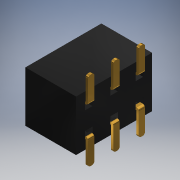
# Autodesk Inventor part: CON-IDC-HE-SMD-2X3-P2MM
Saved by Autodesk Inventor 2018.3 (Build 223284000, 284)
## iProperties
Created: 2020-10-20
Part Number: CON-IDC-HE-SMD-2X3-P2MM
Material: Genérico
Document SubType Name: Modeling
Designer: laguerre
Density: 8.47 g/cm^3
Appearance: Suave - Negro
Author: laguerre
Autodesk Inventor part; units mm, degrees
ref_plane "YZ Plane" through (0, 0, 0) normal (1, 0, 0) x (0, 1, 0)
ref_plane "XZ Plane" through (0, 0, 0) normal (0, 1, 0) x (-1, 0, 0)
ref_plane "XY Plane" through (0, 0, 0) normal (0, 0, 1) x (1, 0, 0)
sketch "Boceto39" plane through (0, 0, 0) normal (0, 0, 1) x (1, 0, 0)
  line L0 (-1, 2) -> (1, 2)
  line L1 (1, 2) -> (1, -2)
  line L2 (1, -2) -> (-1, -2)
  line L3 (-1, -2) -> (-1, 2)
  point P0 (0, 0)
  point P1 (0, 2)
  point P2 (-1, 0)
  dimension "d373" = 4
  dimension "d374" = 2
  constraints: 8 end point, 2 midpoint, 2 parallel, 1 horizontal, 1 horizontal alignment, 1 perpendicular, 1 vertical alignment
  measures "d373" distance of L2.end L0.start
  measures "d374" distance of L0.start L0.end
extrude "Extrusión13" add sketch "Boceto39" along normal blind 4
sketch "Boceto41" plane through (0, 0, 4) normal (0, 0, 1) x (1, 0, 0)
  line L0 (1, 2) -> (-1, 2) projected
  line L1 (-1, 2) -> (-1, -2) projected
  line L2 (-1, -2) -> (1, -2) projected
  line L3 (1, -2) -> (1, 2) projected
  line L4 (-0.3, 1.3) -> (0.3, 1.3)
  line L5 (0.3, 1.3) -> (0.3, 0.7)
  line L6 (0.3, 0.7) -> (-0.3, 0.7)
  line L7 (-0.3, 0.7) -> (-0.3, 1.3)
  line L8 (-0.3, -0.7) -> (0.3, -0.7)
  line L9 (0.3, -0.7) -> (0.3, -1.3)
  line L10 (0.3, -1.3) -> (-0.3, -1.3)
  line L11 (-0.3, -1.3) -> (-0.3, -0.7)
  line L12 (-0.3, 1) -> (0.3, 1) construction
  line L13 (0.3, -1) -> (-0.3, -1) construction
  line L14 (1, 2) -> (-1, 2) projected
  line L15 (-1, -2) -> (1, -2) projected
  point P0 (0, 0)
  point P1 (0, -0.7)
  point P2 (0, 0.7)
  dimension "d384" = 2
  dimension "d387" = 1
  dimension "d390" = 0.6
  constraints: 20 end point, 6 midpoint, 4 parallel, 3 equal length, 2 horizontal, 2 perpendicular, 2 vertical alignment, 1 point on line
  measures "d384" distance between parallel lines of L12 L13
  measures "d387" distance from line of L12 point (0, 0)
  measures "d390" distance of L4.start L4.end
extrude "Extrusión14" cut sketch "Boceto41" against normal blind 4 contours L4 L5 L6 L7 | L8 L9 L10 L11
chamfer "Chaflán5" distance 0.2 angle 45 8 edges at (-0.3, 1, 4) (0, 1.3, 4) (0.3, 1, 4) (0, 0.7, 4) (0, -0.7, 4) (-0.3, -1, 4) (0, -1.3, 4) (0.3, -1, 4)
sketch "Boceto42" plane through (0, 0, 0) normal (1, 0, 0) x (0, 1, 0)
  line L0 (-2, 0) -> (2, 0) construction
  line L1 (1.3, 0) -> (0.7, 0) construction
  line L2 (1.3, 3.8) -> (1.3, 0) projected
  line L3 (1.3, 0.2) -> (1.3, 0)
  line L4 (1.3, 0) -> (3.125, 0)
  line L5 (3.125, 0) -> (3.125, -0.2)
  line L6 (3.125, -0.2) -> (1.3, -0.2)
  line L7 (1.1, 0) -> (1.1, 0.2)
  line L8 (1.1, 0.2) -> (1.3, 0.2)
  arc A0 (1.1, 0) -> (1.3, -0.2) centre (1.3, 0) ccw
  line L9 (-1.3, 0.2) -> (-1.3, 0)
  line L10 (-1.3, 3.8) -> (-1.3, 0) projected
  line L11 (-1.3, 0) -> (-3.125, 0)
  line L12 (-3.125, 0) -> (-3.125, -0.2)
  line L13 (-3.125, -0.2) -> (-1.3, -0.2)
  line L14 (-1.1, 0) -> (-1.1, 0.2)
  line L15 (-1.1, 0.2) -> (-1.3, 0.2)
  arc A1 (-1.3, -0.2) -> (-1.1, 0) centre (-1.3, 0) ccw
  point P0 (0, 0)
  dimension "d401" = 0.2
  dimension "d402" = 0.2
  dimension "d403" = 0.2
  dimension "d404" = 0.2
  dimension "d405" = 6.25
  dimension "d406" = 3.125
  dimension "d407" = 0.2
  constraints: 24 end point, 8 perpendicular, 6 collinear, 4 point on circle, 4 tangent, 2 centre point, 2 equal length, 2 horizontal, 1 point on line
  measures "d401" distance of L4.end L5.end
  measures "d402" radius of A0
  measures "d403" distance of L7.end L3.start
  measures "d404" radius of A1
  measures "d405" distance between parallel lines of L5 L12
  measures "d406" distance from line of point (0, 0) L12
  measures "d407" distance between parallel lines of L0 L15
extrude "Extrusión15" add sketch "Boceto42" along normal mid plane 0.5 separate body
fillet "Empalme44" radius 0.2 4 edges at (0.25, -3.125, -0.1) (-0.25, -3.125, -0.1) (0.25, 3.125, -0.1) (-0.25, 3.125, -0.1)
pattern_linear "Patrón rectangular1" count 3 spacing 2 along (1, 0, 0) of "Extrusión13", "Extrusión14", "Chaflán5", "Extrusión15", "Empalme44" bodies 1
